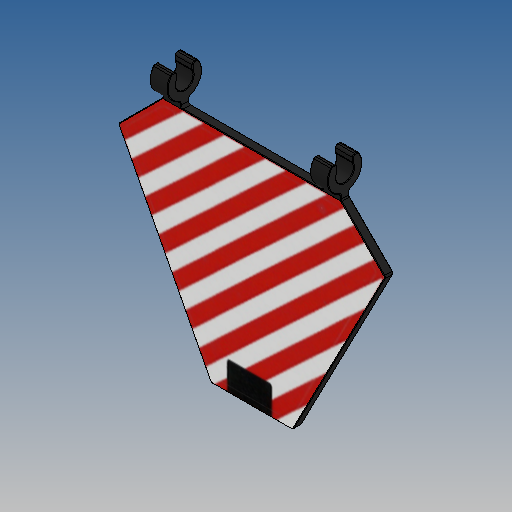
# Autodesk Inventor part: 42146_53913_1
Saved by Autodesk Inventor 2025.1 (Build 291241000, 241)
## iProperties
Created: 2024-12-15
Part Number: 42146_53913_1
Material: ABS-Kunststoff
Document SubType Name: Modeling
Designer: hp.muther
Density: 1.06 g/cm^3
Appearance: Black
Author: hp.muther
Autodesk Inventor part; units mm, degrees
ref_plane "YZ Plane" through (0, 0, 0) normal (1, 0, 0) x (0, 1, 0)
ref_plane "XZ Plane" through (0, 0, 0) normal (0, 1, 0) x (-1, 0, 0)
ref_plane "XY Plane" through (0, 0, 0) normal (0, 0, 1) x (1, 0, 0)
sketch "Skizze1" plane through (0, 0, 0) normal (0, 1, 0) x (-1, 0, 0)
  line L0 (0, -4) -> (16, -4)
  line L1 (16, -4) -> (24, -12)
  line L2 (24, -12) -> (7.3419, -44)
  line L3 (7.3419, -44) -> (0, -44)
  line L4 (0, -44) -> (0, -4)
  point P0 (0, 0)
  dimension "d0" = 40
  dimension "d1" = 24
  dimension "d2" = 16
  dimension "d3" = 4
  dimension "d5" = 45
  dimension "d6" = 27.5
  dimension "d7" = 7.3418
  constraints: 10 end point, 1 horizontal, 1 parallel, 1 perpendicular, 1 point on line
  measures "d0" distance of L3.end L0.start
  measures "d1" distance from line of L1.end L4
  measures "d2" distance from line of L4 L0.end
  measures "d3" distance from line of point (0, 0) L0
  measures "d5" angle of L0 L1
  measures "d6" angle of L4 L2
  measures "d7" distance of L2.end L3.end
extrude "Extrusion1" add sketch "Skizze1" along normal mid plane 1.5
sketch "Skizze2" plane through (0, -0.75, -44) normal (1, 0, 0) x (0, 0, -1)
  line L0 (-40, 0) -> (-40, 1.5) projected
  arc A0 (-44.7746, -0.65) -> (-44.7746, 2.15) centre (-44, 0.75) ccw
  line L1 (-44.7746, -0.65) -> (-46, -0.65)
  line L2 (-46, -0.65) -> (-46, -1.6185)
  line L3 (-44.7746, 2.15) -> (-46, 2.15)
  line L4 (-46, 2.15) -> (-46, 3.1185)
  arc A1 (-46, -1.6185) -> (-46, 3.1185) centre (-44, 0.75) ccw
  line L5 (-40, 0) -> (-40.9921, 0)
  line L6 (-40, 1.5) -> (-40.9921, 1.5)
  dimension "d10" = 3.2
  dimension "d11" = 6.2
  dimension "d12" = 6
  dimension "d13" = 2.8
  constraints: 12 end point, 6 point on circle, 3 horizontal, 2 centre point, 2 coincident, 2 parallel, 2 perpendicular, 1 collinear
  measures "d10" diameter of A0
  measures "d11" diameter of A1
  measures "d12" distance between parallel lines of L2 L0
  measures "d13" distance between parallel lines of L3 L1
extrude "Extrusion2" add sketch "Skizze2" against normal blind 16
fillet "Rundung1" radius 0.4 11 edges at (-8, -0.75, -3.0079) (-8, 0.75, -3.0079) (-8, -1.4, 0.7746) (-8, 1.4, 0.7746) (-8, -1.4, 2) (-8, 2.3685, 2) (-8, 1.4, 2) (-8, -2.3685, 2) (-7.3419, 0, -44) (-24, 0, -12) (-16, 0, -4)
fillet "Rundung1" radius 0.1 15 edges at (-3.6709, 0.75, -44) (-15.6709, 0.75, -28) (-15.6709, -0.75, -28) (-3.6709, -0.75, -44) (-20, 0.75, -8) (-20, -0.75, -8) (-16, -0.75, -3.504) (-16, 0.75, -3.504) (-16, -2.9498, -0.9534) (-16, 0, -1.6) (-16, -1.4, 1.3873) (-16, 1.4, 1.3873) (-16, 1.8843, 2) (-16, 2.9498, -0.9534) (-16, -1.8843, 2)
sketch "Skizze3" plane through (0, 0, 0) normal (0, 1, 0) x (-1, 0, 0)
  line L0 (0, -43.9) -> (0, -3.3057) projected
  line L1 (0, -4) -> (12.8, -4)
  line L2 (12.8, -4) -> (12.8, 2)
  line L3 (12.8, 2) -> (0, 2)
  line L4 (0, 2) -> (0, -4)
  line L5 (15.9, 2) -> (0, 2) projected
  line L6 (16, 0.8718) -> (16, 1.6) projected
  point P0 (0, 0)
  point P1 (0, -3.3057)
  dimension "d18" = 4
  dimension "d19" = 3.2
  constraints: 8 end point, 2 parallel, 1 collinear, 1 horizontal, 1 perpendicular, 1 point on line
  measures "d18" distance from line of L1 point (0, 0)
  measures "d19" distance between parallel lines of L2 L6
extrude "Extrusion3" cut sketch "Skizze3" along normal through all both and the other way through all
fillet "Rundung2" radius 0.1 17 edges at (-12.8, -0.824, -3.0739) (-12.8, -2.9607, -0.9187) (-12.8, -2.3554, 1.9569) (-12.8, -1.9874, 2) (-12.8, -1.5172, 1.8828) (-12.8, -1.4, 1.2359) (-12.8, -1.4101, 0.7823) (-12.8, 0, -1.6) (-12.8, 1.4101, 0.7823) (-12.8, 1.4, 1.2359) (-12.8, 1.5172, 1.8828) (-12.8, 1.9874, 2) (-12.8, 2.3554, 1.9569) (-12.8, 2.9607, -0.9187) (-12.8, 0.824, -3.0739) (-6.4, -0.75, -4) (-6.4, 0.75, -4)
fillet "Rundung2" radius 0.4 1 edges at (-12.8, 0, -4)
mirror "Spiegeln1" about plane through (0, 0, -4) normal (1, 0, 0)
sketch "Skizze5" plane through (0, -0.75, 0) normal (0, -1, 0) x (1, 0, 0)
  arc A0 (-16.0464, -4.1879) -> (-15.9, -3.8343) centre (-16.4, -3.8343) ccw projected
  line L0 (-23.7219, -11.8633) -> (-16.0464, -4.1879) projected
  arc A1 (-23.7219, -11.8633) -> (-23.7759, -12.214) centre (-23.5098, -12.0755) ccw projected
  line L1 (-7.3652, -43.7385) -> (-23.7759, -12.214) projected
  arc A2 (-7.3652, -43.7385) -> (-7.0991, -43.9) centre (-7.0991, -43.6) ccw projected
  line L2 (-7.0991, -43.9) -> (7.0991, -43.9) projected
  arc A3 (7.0991, -43.9) -> (7.3652, -43.7385) centre (7.0991, -43.6) ccw projected
  line L3 (7.3652, -43.7385) -> (23.7759, -12.214) projected
  arc A4 (23.7759, -12.214) -> (23.7219, -11.8633) centre (23.5098, -12.0755) ccw projected
  line L4 (23.7219, -11.8633) -> (16.0464, -4.1879) projected
  arc A5 (15.9, -3.8343) -> (16.0464, -4.1879) centre (16.4, -3.8343) ccw projected
  line L5 (15.9, -3.8343) -> (15.9, -3.3057) projected
  line L6 (15.9, -3.3057) -> (12.9, -3.3057) projected
  line L7 (12.9, -3.3057) -> (12.9, -3.6) projected
  arc A6 (12.4, -4.1) -> (12.9, -3.6) centre (12.4, -3.6) ccw projected
  line L8 (12.4, -4.1) -> (-12.4, -4.1) projected
  line L9 (-12.4, -4.1) -> (-15.9764, -4.1)
  line L10 (12.4, -4.1) -> (12.4, -4) projected
  line L11 (12.4, -4.1) -> (15.9764, -4.1)
  line L12 (12.9, -3.3057) -> (15.9, -3.3057) projected
  point P0 (0, 0)
  constraints: 4 end point, 2 point on circle, 1 horizontal, 1 parallel
extrude "Extrusion4" add sketch "Skizze5" along normal blind 0.01 contours A0 L9 L8 L11 A5 L4 A4 L3 A3 L2 A2 L1 A1 L0
sketch "Skizze6" plane through (0, 0.75, 0) normal (0, 1, 0) x (1, 0, 0)
  line L0 (12.4, 4.1) -> (-12.4, 4.1) projected
  arc A0 (16.0464, 4.1879) -> (15.9, 3.8343) centre (16.4, 3.8343) ccw projected
  line L1 (16.0464, 4.1879) -> (23.7219, 11.8633) projected
  arc A1 (23.7219, 11.8633) -> (23.7759, 12.214) centre (23.5098, 12.0755) ccw projected
  line L2 (23.7759, 12.214) -> (7.3652, 43.7385) projected
  arc A2 (7.3652, 43.7385) -> (7.0991, 43.9) centre (7.0991, 43.6) ccw projected
  line L3 (-7.0991, 43.9) -> (7.0991, 43.9) projected
  arc A3 (-7.0991, 43.9) -> (-7.3652, 43.7385) centre (-7.0991, 43.6) ccw projected
  line L4 (-23.7759, 12.214) -> (-7.3652, 43.7385) projected
  arc A4 (-23.7759, 12.214) -> (-23.7219, 11.8633) centre (-23.5098, 12.0755) ccw projected
  line L5 (-16.0464, 4.1879) -> (-23.7219, 11.8633) projected
  arc A5 (-15.9, 3.8343) -> (-16.0464, 4.1879) centre (-16.4, 3.8343) ccw projected
  line L6 (12.4, 4.1) -> (15.9764, 4.1)
  line L7 (16, 3.8343) -> (15.9, 3.8343) projected
  line L8 (-12.4, 4.1) -> (-15.9764, 4.1)
  point P0 (0, 0)
  constraints: 4 end point, 2 point on circle, 1 collinear, 1 parallel
extrude "Extrusion5" add sketch "Skizze6" along normal blind 0.01
sketch "Skizze4" plane through (0, -0.76, 0) normal (0, -1, 0) x (1, 0, 0)
  line L0 (-25.5, -86.5655) -> (-25.5, -2.6) construction
  line L1 (-25.5, -2.6) -> (24.5, -2.6) construction
  line L2 (24.5, -2.6) -> (24.5, -86.5655) construction
  line L3 (24.5, -86.5655) -> (-25.5, -86.5655) construction
  line L4 (15.9764, -4.1) -> (-15.9764, -4.1) projected
  point P0 (0, -4.1)
  dimension "d40" = 50
  dimension "d46" = 1.5
  dimension "d51" = 25.5
  constraints: 1 midpoint, 2 other
  measures "d40" distance of L0.end L1.end
  measures "d46" distance between parallel lines of L1 L4
  measures "d51" distance from line of point (0, -4.1) L0
decal "Aufkleber1"
sketch "Skizze7" plane through (0, 0.76, 0) normal (0, 1, 0) x (1, 0, 0)
  line L0 (-15.9764, 4.1) -> (15.9764, 4.1) projected
  line L1 (-25.5, 2.1) -> (-25.5, 86.0655) construction
  line L2 (-25.5, 86.0655) -> (24.5, 86.0655) construction
  line L3 (24.5, 86.0655) -> (24.5, 2.1) construction
  line L4 (24.5, 2.1) -> (-25.5, 2.1) construction
  point P0 (0, 0)
  dimension "d57" = 2
  dimension "d58" = 50
  dimension "d61" = 24.5
  constraints: 1 parallel, 2 other
  measures "d57" distance between parallel lines of L4 L0
  measures "d58" distance of L3.end L1.start
  measures "d61" distance from line of point (0, 0) L3
decal "Aufkleber2"
